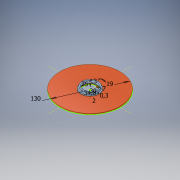
# Autodesk Inventor part: Stewart-Plate-Head
Saved by Autodesk Inventor 2018.3 (Build 223284000, 284)
## iProperties
Created: 2018-02-18
Part Number: Stewart-Plate-Head
Material: Generisch
Document SubType Name: Modeling
Designer: JochenAlt
Density: 1 g/cm^3
Appearance: Vorgabe
Author: JochenAlt
Autodesk Inventor part; units mm, degrees
ref_plane "YZ Plane" through (0, 0, 0) normal (1, 0, 0) x (0, 1, 0)
ref_plane "XZ Plane" through (0, 0, 0) normal (0, 1, 0) x (-1, 0, 0)
ref_plane "XY Plane" through (0, 0, 0) normal (0, 0, 1) x (1, 0, 0)
sketch "Skizze1" plane through (0, 0, 0) normal (0, 0, 1) x (1, 0, 0)
  line L0 (-91, 0) -> (91, 0) construction
  circle A0 centre (0, 0) radius 65
  line L1 (-9.5, 25) -> (9.5, 25)
  line L2 (9.5, 25) -> (9.5, 22)
  line L3 (9.5, 22) -> (-9.5, 22)
  line L4 (-9.5, 22) -> (-9.5, 25)
  line L5 (1.5, 22) -> (-1.5, 22)
  line L6 (-1.5, 22) -> (-1.5, 15)
  line L7 (-1.5, 15) -> (1.5, 15)
  line L8 (1.5, 15) -> (1.5, 22)
  circle A1 centre (0, 0) radius 15
  line L9 (0, 91) -> (0, -91) construction
  circle A2 centre (0, 0) radius 17.4
  circle A3 centre (0, 0) radius 19.4
  circle A4 centre (0, 0) radius 19.7
  dimension "d9" = 130
  dimension "d10" = 3
  dimension "d14" = 19
  dimension "d23" = 7
  dimension "d62" = 30
  dimension "d149" = 25
  dimension "d157" = 34.8
  dimension "d163" = 2
  dimension "d168" = 0.3
  constraints: 16 end point, 5 centre point, 4 coincident, 4 parallel, 3 perpendicular, 2 horizontal, 1 midpoint, 1 point on line, 1 other
  measures "d9" diameter of A0
  measures "d10" distance between parallel lines of L3 L1
  measures "d14" distance between parallel lines of L2 L4
  measures "d23" distance between parallel lines of L3 L7
  measures "d62" diameter of A1
  measures "d149" distance from line of A0.centre L1
  measures "d157" diameter of A2
  measures "d163" radial gap between concentric circles of A3 A2
  measures "d168" radial gap between concentric circles of A4 A3
extrude "Extrusion3" add sketch "Skizze1" against normal blind 8 contours L1 L2 L3 L4 | L3 L8 A4 L6 | A4 L8 A3 L6 | A3 L8 A2 L6 | A2 L8 L7 L6 picked at (1.1668, 19.4594) picked at (-1.1669, 18.0233) picked at (-0.6669, 15.7976)
chamfer "Fase2" distance 3 distance2 8 1 edges at (-9.5, 23.5, -8) measured on face at (-9, 23.5, -8)
chamfer "Fase3" distance 3 distance2 8 1 edges at (9.5, 23.5, -8) measured on face at (9, 23.5, -8)
fillet "Rundung1" radius 4 2 edges at (-6.5001, 23.5, -8) (6.5001, 23.5, -8)
sketch "Skizze2" plane through (-9.5, 25, 0) normal (0, 1, 0) x (1, 0, 0)
  circle A0 centre (6, 4.5) radius 0.9
  circle A1 centre (13, 4.5) radius 0.9
  line L0 (43, 0) -> (-27, 0) construction
  line L1 (-1.6221, 4.5) -> (19.0112, 4.5) construction
  line L2 (3, 8) -> (16, 8) construction
  line L3 (0, 0) -> (0, 1) projected
  line L4 (9.5, 9.6) -> (9.5, -1.6) construction
  point P0 (9.5, 0)
  point P1 (4, 7)
  point P2 (11, 7)
  point P3 (0, 3)
  dimension "d16" = 1.8
  dimension "d20" = 3.5
  dimension "d150" = 7
  constraints: 2 centre point, 2 end point, 1 equal radius, 1 horizontal, 1 point on line, 1 symmetric about line, 1 other
  measures "d16" diameter of A0
  measures "d150" distance of A1.centre A0.centre
extrude "Extrusion4" cut sketch "Skizze2" against normal up to next
chamfer "Fase1" distance 7 distance2 5 1 edges at (0, 15, -8) measured on face at (0, 15.5, -8)
pattern_circular "Runde Anordnung1" count 3 over 360 about axis through (0, 0, -10) along (0, 0, 1) of "Extrusion4", "Extrusion3", "Fase2", "Fase3", "Rundung1", "Fase1"
extrude "Extrusion11" add sketch "Skizze1" along normal blind 2 contours A0 | L1 L2 L3 L4 | L3 L8 A4 L6 | A4 L8 A3 L6 | L6 A3 L8 A4 | A3 L8 A2 L6 | L6 A2 L8 A3 | A2 L8 L7 L6 | L6 L7 L8 A2
extrude "Extrusion14" cut sketch "Skizze1" against normal blind 0.5 from surface at 2 contours A4 L8 A3 L6 | L6 A3 L8 A4 | A3 L8 A2 L6 | L6 A2 L8 A3 | A2 L8 L7 L6 | L6 L7 L8 A2
extrude "Extrusion12" add sketch "Skizze1" along normal blind 6 from surface at 2 separate body contours A2 L8 L7 L6 | L6 L7 L8 A2
chamfer "Fase4" distance 0.5 angle 45 1 edges at (-17.4, 0, 8)
extrude "Extrusion13" add sketch "Skizze1" along normal blind 1 from surface at 2 contours A3 L8 A2 L6 | L6 A2 L8 A3 | A2 L8 L7 L6 | L6 L7 L8 A2 bodies 2
